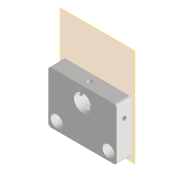
# Autodesk Inventor part: Anglerfish_coverslipclamp_lampclamp
Saved by Autodesk Inventor 2022 (Build 260153000, 153)
## iProperties
Created: 2023-04-17
Part Number: Anglerfish_coverslipclamp_lampclamp
Material: Generisch
Document SubType Name: Modeling
Designer: diederichbenedict
Density: 1 g/cm^3
Appearance: Vorgabe
Author: diederichbenedict
Autodesk Inventor part; units mm, degrees
ref_plane "YZ Plane" through (0, 0, 0) normal (1, 0, 0) x (0, 1, 0)
ref_plane "XZ Plane" through (0, 0, 0) normal (0, 1, 0) x (-1, 0, 0)
ref_plane "XY Plane" through (0, 0, 0) normal (0, 0, 1) x (1, 0, 0)
ref_plane "Arbeitsebene1" through (0, 0, 0) normal (0, 0, 1) x (1, 0, 0)
sketch "Skizze1" plane through (0, 0, 0) normal (0, 0, 1) x (1, 0, 0)
  circle A0 centre (17.3893, 23.3893) radius 1.4 projected
  circle A1 centre (-17.3893, -25.3893) radius 1.4 projected
  circle A2 centre (17.3893, -25.3893) radius 1.4 projected
  circle A3 centre (-17.3893, 23.3893) radius 1.4 projected
  arc A4 (21, -31) -> (23, -29) centre (21, -29) ccw projected
  line L0 (23, -29) -> (23, 29) projected
  line L1 (11.5, 29) -> (23, 29) projected
  line L2 (11.5, 29) -> (11.5, -19) projected
  line L3 (11.5, -19) -> (-11.5, -19) projected
  line L4 (-11.5, -19) -> (-11.5, 29) projected
  line L5 (-23, 29) -> (-11.5, 29) projected
  line L6 (-23, 29) -> (-23, -29) projected
  arc A5 (-23, -29) -> (-21, -31) centre (-21, -29) ccw projected
  line L7 (-21, -31) -> (21, -31) projected
  circle A6 centre (-17.3893, -25.3893) radius 4
  circle A7 centre (17.3893, -25.3893) radius 4
  line L8 (-21, -31) -> (21, -31)
  line L9 (23, -29) -> (23, 2)
  line L10 (21, 4) -> (-21, 4)
  line L11 (-23, 2) -> (-23, -29)
  circle A8 centre (0, -6) radius 5.75
  arc A9 (-21, 4) -> (-23, 2) centre (-21, 2) ccw
  arc A10 (23, 2) -> (21, 4) centre (21, 2) ccw
  arc A11 (21, -31) -> (23, -29) centre (21, -29) ccw
  arc A12 (-23, -29) -> (-21, -31) centre (-21, -29) ccw
  point P0 (0, 0)
  point P1 (23, 4)
  dimension "d0" = 8
  dimension "d1" = 8
  dimension "d2" = 11.5
  dimension "d3" = 25
  dimension "d4" = 35
  dimension "d5" = 0
  dimension "d6" = 2
  constraints: 8 end point, 8 point on circle, 8 tangent, 7 centre point, 3 equal radius, 3 point on line, 2 coincident, 2 parallel, 1 horizontal, 1 perpendicular
  measures "d0" diameter of A6
  measures "d1" diameter of A7
  measures "d2" diameter of A8
  measures "d3" distance from line of A8.centre L7
  measures "d4" distance between parallel lines of L10 L7
  measures "d5" distance between parallel lines of L7 L8
  measures "d6" radius of A9
extrude "Extrusion1" add sketch "Skizze1" along normal blind 10 contours L7 A5 L6 A9 L10 L4 L3 L2 A10 L0 A4 | L2 L3 L4 L10
sketch "Skizze2" plane through (23, -29, 0) normal (1, 0, 0) x (0, 0, -1)
  line L0 (-10, 17.25) -> (0, 17.25) projected
  line L1 (-10, 28.75) -> (0, 28.75) projected
  line L2 (-10, 0) -> (-10, 31) projected
  line L3 (0, 0) -> (0, 31) projected
  circle A0 centre (-5, 23) radius 1.4
  point P0 (0, 29)
  dimension "d9" = 2.8
  dimension "d10" = 5.75
  constraints: 1 centre point
  measures "d9" diameter of A0
  measures "d10" distance from line of A0.centre L0
extrude "Extrusion2" cut sketch "Skizze2" against normal through all contours A0
sketch "Skizze3" plane through (-21, -31, 0) normal (0, -1, 0) x (1, 0, 0)
  line L0 (15.25, 10) -> (15.25, 0) projected
  line L1 (26.75, 10) -> (26.75, 0) projected
  circle A0 centre (21, 5) radius 1.4
  point P0 (21, 0)
  dimension "d13" = 2.8
  constraints: 1 centre point
  measures "d13" diameter of A0
extrude "Extrusion3" cut sketch "Skizze3" against normal through all
